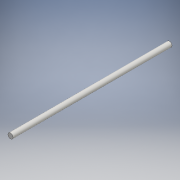
# Autodesk Inventor part: palo
Saved by Autodesk Inventor 2016 (Build 200138000, 138)
## iProperties
Created: 2016-02-19
Part Number: palo
Material: Genérico
Document SubType Name: Modeling
Designer: Usuario1
Density: 1 g/cm^3
Appearance: Valor por defecto
Author: Usuario1
Autodesk Inventor part; units mm, degrees
ref_plane "YZ Plane" through (0, 0, 0) normal (1, 0, 0) x (0, 1, 0)
ref_plane "XZ Plane" through (0, 0, 0) normal (0, 1, 0) x (-1, 0, 0)
ref_plane "XY Plane" through (0, 0, 0) normal (0, 0, 1) x (1, 0, 0)
sketch "Boceto1" plane through (0, 0, 0) normal (0, 0, 1) x (1, 0, 0)
  line L0 (0, 0) -> (0, 24.984)
  line L1 (0.4, 24.984) -> (0.4, 0)
  line L2 (0.4, 0) -> (0, 0)
  line L3 (0, 24.984) -> (0.4, 24.984)
  constraints: 8 end point
revolve "Revolución1" add sketch "Boceto1" angle 360 about axis through (0, 0, 0) along (0, 1, 0)
